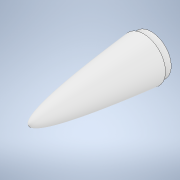
# Autodesk Inventor part: nose-basepart1
Saved by Autodesk Inventor 2020.3 (Build 243373000, 373)
## iProperties
Created: 2021-03-10
Part Number: nose-basepart1
Material: ABS Plastic
Document SubType Name: Modeling
Designer: 0x6f736f646f
Density: 1.06 g/cm^3
Appearance: Smooth - White
Mass: 17.0739 g
Surface Area: 229.369 cm^2
Volume: 17.0739 cm^3
Author: 0x6f736f646f
Autodesk Inventor part; units mm, degrees
ref_plane "YZ Plane" through (0, 0, 0) normal (1, 0, 0) x (0, 1, 0)
ref_plane "XZ Plane" through (0, 0, 0) normal (0, 1, 0) x (-1, 0, 0)
ref_plane "XY Plane" through (0, 0, 0) normal (0, 0, 1) x (1, 0, 0)
sketch "Sketch2" plane through (0, 0, 0) normal (1, 0, 0) x (0, 1, 0)
  line L0 (0, 0) -> (26, 0)
  line L1 (26, 0) -> (26, -10)
  line L2 (0, 2) -> (23.5, 2)
  line L3 (0, 0) -> (-26, 0)
  line L4 (-26, 0) -> (-26, -10)
  line L5 (0, 2) -> (-23.5, 2)
  line L6 (0, 0) -> (0, 212.5)
  line L7 (0, 0) -> (0, 150)
  line L8 (23.5, 2) -> (23.5, 0)
  line L9 (-23.5, 2) -> (-23.5, 0)
  line L10 (0, 0) -> (0, 145)
  spline S0 degree 2 poles (28.5, 0) (0, 300) (-28.5, 0) knots 0 0 0 1 1 1
  spline S1 degree 2 poles (23.5, 0) (0, 290) (-23.5, 0) knots 0 0 0 1 1 1
  line L11 (0, 2) -> (-7.0238, 2)
  line L12 (0, 172) -> (0, 2)
  line L13 (0, 0) -> (-5, 0)
  line L14 (0, 212.5) -> (0, 0)
  line L15 (-7.0238, 2) -> (-15.0238, 2)
  line L16 (-23.5, 2) -> (-28.3094, 2)
  line L17 (0, -54.5) -> (0, 257) projected
  line L18 (23.5, 0) -> (23.5, -10)
  line L19 (23.5, -10) -> (26, -10)
  line L20 (-23.5, 0) -> (-23.5, -10)
  line L21 (-23.5, -10) -> (-26, -10)
  line L22 (28.5, 0) -> (26, 0)
  line L23 (-26, 0) -> (-28.5, 0)
  point P0 (0.3832, 149.9729)
  point P1 (28.3225, 1.8623)
  point P2 (23.3374, 2)
  point P3 (0, 2)
  point P4 (3, 2)
  point P5 (-23.3374, 2)
  dimension "d51" = 26
  dimension "d54" = 2
  dimension "d55" = 26
  dimension "d59" = 150
  dimension "d60" = 23.5
  dimension "d61" = 23.5
  dimension "d62" = 145
  dimension "d64" = 23.5
  dimension "d80" = 5
  dimension "d81" = 10
  dimension "d82" = 5
  dimension "d83" = 10
  constraints: 46 end point, 8 horizontal, 8 point on line, 6 perpendicular, 2 equal length, 2 vertical, 9 other
  measures "d51" distance of L0.start L0.end
  measures "d54" distance between parallel lines of L0 L2
  measures "d55" distance of L0.start L3.end
  measures "d59" distance of L0.start L7.end
  measures "d60" distance of L2.start L2.end
  measures "d61" distance of L2.start L5.end
  measures "d62" distance of L0.start L10.end
  measures "d64" distance between parallel lines of L6 L8
  measures "d80" distance of L8.end L22.start
  measures "d81" distance between parallel lines of L0 L19
  measures "d82" distance of L23.end L9.end
  measures "d83" distance between parallel lines of L3 L21
revolve "Revolution5" add sketch "Sketch2" angle 360 mid plane about axis through (0, 0, -10) along (0, 0, 1) contours L8 L2 S1 L6 S0 L22 L0 | L0 L1 L19 L18
extrude "Extrusion4" [suppressed]
sketch "Sketch3" plane through (0, 0, 0) normal (0, 1, 0) x (-1, 0, 0)
  circle A0 centre (0, 102.5) radius 2.5
  point P0 (0, 0)
  dimension "d77" = 5
  constraints: 1 centre point
  measures "d77" diameter of A0
extrude "Extrusion5" cut sketch "Sketch3" against normal blind 30
body "Solid4"
